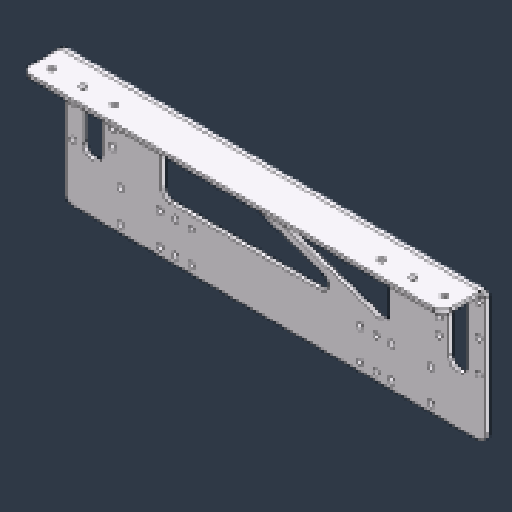
# Autodesk Inventor part: PLATE,MOUNT,DRIVE,ELEVATOR
Saved by Autodesk Inventor 2024.3 (Build 283343000, 343)
## iProperties
Category: _
Manager: _
Created: 2025-01-29
Part Number: PLATE,MOUNT,DRIVE,ELEVATOR
Checked By: 00
Engr Approved By: _
User Status: Work In Process
Material: Sheet Metal, Aluminum, 3003
Description: SHEET METAL (mm)
Document SubType Name: Sheet Metal
Mfg Approved By: John.Thibert
Designer: John.Thibert
Manufacturer: Standard
Standards Organization: Custom
Density: 2.73 g/cm^3
Sheet Metal Rule: Default
Appearance: Metal-AL-6061 (Flat)
Mass: 317.836 g
Surface Area: 810.801 cm^2
Volume: 116.424 cm^3
ILogicPurgeVersion: 2.2.20.20
OnSaveVersion: 3.4.3.0
OnSaveAssembly: COREAutomationManager
CN_MASS: 0.32
CL_runCount: 1
CN_SERVICEABLE: _
FIRST_DESCRIPTION: _
SECOND_DESCRIPTION: _
THIRD_DESCRIPTION: _
ModelCat: Uncategorized
MaterialName: Sheet Metal, Aluminum, 3003
Subject: _
Author: John.Thibert
Keywords: -
Revision Number: A
Autodesk Inventor part; units mm, degrees
ref_plane "YZ Plane" through (0, 0, 0) normal (1, 0, 0) x (0, 1, 0)
ref_plane "XZ Plane" through (0, 0, 0) normal (0, 1, 0) x (-1, 0, 0)
ref_plane "XY Plane" through (0, 0, 0) normal (0, 0, 1) x (1, 0, 0)
sketch "Sketch1" plane through (0, 0, 0) normal (0, 0, 1) x (1, 0, 0)
  line L0 (169.8625, -50.8) -> (-169.8625, -50.8)
  line L1 (-169.8625, -50.8) -> (-169.8625, 50.8)
  line L2 (-169.8625, 50.8) -> (169.8625, 50.8)
  line L3 (169.8625, 50.8) -> (169.8625, -50.8)
  line L4 (169.8625, -50.8) -> (-169.8625, 50.8) construction
  line L5 (-169.8625, -50.8) -> (169.8625, 50.8) construction
  point P0 (0, 0)
  dimension "d0" = 339.725
  dimension "d1" = 101.6
  measures "d0" distance of L1.end L2.end
  measures "d1" distance of L0.end L1.end
extrude "Plate1" add sketch "Sketch1" along normal mid plane 3.175
sketch "Sketch2" plane through (-169.8625, 55.5625, 6.35) normal (0, 1, 0) x (-1, 0, 0)
  line L0 (-339.725, 0) -> (0, 0)
  line L1 (0, 0) -> (0, 30.1625)
  line L2 (0, 30.1625) -> (-339.725, 30.1625)
  line L3 (-339.725, 30.1625) -> (-339.725, 0)
  constraints: 6 end point, 1 horizontal, 1 perpendicular, 1 vertical
edge flange "Flange1" height 38.1 angle 90 thickness 3.175 bend radius 4.7625 thickness toward (0, 1, 0) relief tear relief width 3.175 relief depth 1.5875 edges at (0, 50.8, 1.5875) wall of the first edge with corners at (169.8625, 55.5625, 6.35) (-169.8625, 55.5625, 6.35) (-169.8625, 55.5625, 36.5125) (169.8625, 55.5625, 36.5125)
bend "Bend1"
corner "Corner1"
sketch "Sketch3" plane through (0, 0, 1.5875) normal (0, 0, 1) x (1, 0, 0)
  line L0 (163.5252, -4.7625) -> (-163.5252, -4.7625) construction
  line L1 (-163.5252, -4.7625) -> (-163.5252, 46.0375) construction
  line L2 (-163.5252, 46.0375) -> (163.5252, 46.0375) construction
  line L3 (163.5252, 46.0375) -> (163.5252, -4.7625) construction
  line L4 (163.5252, -4.7625) -> (-163.5252, 46.0375) construction
  line L5 (-163.5252, -4.7625) -> (163.5252, 46.0375) construction
  line L6 (-237.8075, 0) -> (237.8075, 0) construction
  line L7 (0, 80.645) -> (0, -72.7075) construction
  line L8 (169.8625, 58.7375) -> (-169.8625, 58.7375) construction
  point P0 (0, 20.6375)
  point P1 (-163.5252, 20.6375)
  point P2 (163.5252, 20.6375)
  dimension "d13" = 327.0504
  dimension "d14" = 50.8
  dimension "d44" = 12.7
  constraints: 12 end point, 4 coincident, 4 midpoint, 2 parallel, 1 horizontal, 1 perpendicular, 1 point on line
  measures "d13" distance of L1.end L2.end
  measures "d14" distance of L0.end L1.end
  measures "d44" distance between parallel lines of L2 L8
hole "Hole1" at (-163.5252, 46.0375, 1.5875) at (163.5252, 46.0375, 1.5875) at (-163.5252, 20.6375, 1.5875) at (-163.5252, -4.7625, 1.5875) at (163.5252, 20.6375, 1.5875) at (163.5252, -4.7625, 1.5875) direction (0, 0, -1) diameter 5.1054 end through all clearance for "Flat Head Machine Screw (82)" size "#10" standard "Ansi Unified Screw Threads"
sketch "Sketch4" plane through (0, 0, 1.5875) normal (0, 0, 1) x (1, 0, 0)
  line L0 (95.25, -12.7) -> (-95.25, -12.7) construction
  line L1 (-95.25, -12.7) -> (-95.25, 50.8) construction
  line L2 (-95.25, 50.8) -> (95.25, 50.8) construction
  line L3 (95.25, 50.8) -> (95.25, -12.7) construction
  line L4 (95.25, -12.7) -> (-95.25, 50.8) construction
  line L5 (-95.25, -12.7) -> (95.25, 50.8) construction
  line L6 (-75.6848, 47.625) -> (92.075, 47.625)
  line L7 (92.075, 47.625) -> (92.075, -8.2949)
  line L8 (92.075, -8.2949) -> (-75.6848, 47.625)
  line L9 (-92.075, -9.525) -> (75.6848, -9.525)
  line L10 (75.6848, -9.525) -> (-92.075, 46.3949)
  line L11 (-92.075, 46.3949) -> (-92.075, -9.525)
  line L12 (-147.6375, -3.175) -> (-147.6375, 41.275) construction
  line L13 (-155.575, -3.175) -> (-155.575, 41.275)
  line L14 (-139.7, 41.275) -> (-139.7, -3.175)
  arc A0 (-155.575, -3.175) -> (-139.7, -3.175) centre (-147.6375, -3.175) ccw
  arc A1 (-139.7, 41.275) -> (-155.575, 41.275) centre (-147.6375, 41.275) ccw
  line L15 (0, 80.645) -> (0, -72.7075) construction
  line L16 (147.6375, -3.175) -> (147.6375, 41.275) construction
  line L17 (155.575, -3.175) -> (155.575, 41.275)
  line L18 (139.7, 41.275) -> (139.7, -3.175)
  arc A2 (139.7, -3.175) -> (155.575, -3.175) centre (147.6375, -3.175) ccw
  arc A3 (155.575, 41.275) -> (139.7, 41.275) centre (147.6375, 41.275) ccw
  line L19 (-147.6375, 19.05) -> (147.6375, 19.05) construction
  line L20 (-237.8075, 0) -> (237.8075, 0) construction
  line L21 (169.8625, 58.7375) -> (-169.8625, 58.7375) construction
  point P0 (0, 19.05)
  dimension "d22" = 63.5
  dimension "d23" = 190.5
  dimension "d24" = 3.175
  dimension "d25" = 3.175
  dimension "d29" = 7.9375
  dimension "d30" = 44.45
  dimension "d31" = 147.6375
  dimension "d45" = 39.6875
  constraints: 42 end point, 8 point on circle, 7 symmetric about line, 4 centre point, 4 midpoint, 4 tangent, 3 parallel, 3 perpendicular, 1 horizontal, 1 horizontal alignment, 1 vertical, 6 other
  measures "d22" distance of L0.end L1.end
  measures "d23" distance of L1.end L2.end
  measures "d24" distance between parallel lines of L0 L9
  measures "d25" distance between parallel lines of L2 L6
  measures "d29" radius of A1
  measures "d30" distance of L12.start L12.end
  measures "d31" distance between parallel lines of L12 L15
  measures "d45" distance between parallel lines of L19 L21
extrude "Cut1" cut sketch "Sketch4" against normal through all
sketch "Sketch6" plane through (0, 0, 1.5875) normal (0, 0, 1) x (1, 0, 0)
  line L0 (-93.6625, -19.05) -> (-93.6625, -44.45) construction
  line L1 (-169.8625, -50.8) -> (-169.8625, 50.8) construction
  point P0 (0, 0)
  dimension "d46" = 25.4
  dimension "d47" = 76.2
  dimension "d58" = 19.05
  constraints: 2 coincident, 2 end point, 1 vertical
  measures "d46" distance of L0.start L0.end
  measures "d47" distance between parallel lines of L1 L0
  measures "d58" vertical distance of point (-93.663, -19.05) point (0, 0)
hole "Hole2" at (-93.6625, -19.05, 1.5875) at (-93.6625, -44.45, 1.5875) direction (0, 0, -1) diameter 5.1054 end through all clearance for "Flat Head Machine Screw (82)" size "#10" standard "Ansi Unified Screw Threads"
pattern_linear "Rectangular Pattern1" count 2 spacing 31.75 along (-1, 0, 0) of "Hole2"
pattern_linear "Rectangular Pattern2" count 3 spacing 12.7 along (1, 0, 0) of "Hole2"
sketch "Sketch7" plane through (0, 0, 1.5875) normal (0, 0, 1) x (1, 0, 0)
  line L0 (-139.7, 41.275) -> (-139.7, -3.175) construction
  line L1 (-131.7625, 31.8516) -> (-131.7625, 6.4516) construction
  point P0 (0, 0)
  point P1 (-131.7625, 19.1516)
  dimension "d62" = 25.4
  dimension "d63" = 7.9375
  dimension "d64" = 19.1516
  constraints: 2 coincident, 2 end point, 1 midpoint, 1 vertical
  measures "d62" distance of L1.start L1.end
  measures "d63" distance between parallel lines of L0 L1
  measures "d64" vertical distance of point (0, 0) point (-131.763, 19.152)
hole "Hole3" at (-131.7625, 31.8516, 1.5875) at (-131.7625, 19.1516, 1.5875) at (-131.7625, 6.4516, 1.5875) direction (0, 0, -1) diameter 5.1054 end through all clearance for "Flat Head Machine Screw (82)" size "#10" standard "Ansi Unified Screw Threads"
sketch "Sketch8" plane through (-169.8625, 55.5625, 6.35) normal (0, -1, 0) x (1, 0, 0)
  line L0 (0, -4.7625) -> (339.725, -4.7625) construction
  line L1 (0, 30.1625) -> (0, 0) construction
  point P0 (169.8625, -6.35)
  point P1 (11.1125, 17.4625)
  dimension "d72" = 22.225
  dimension "d73" = 11.1125
  measures "d72" distance from line of point (11.113, 17.462) L0
  measures "d73" distance from line of point (11.113, 17.462) L1
mirror "Mirror1" about plane through (0, 0, 0) normal (1, 0, 0) of "Hole2", "Rectangular Pattern1", "Rectangular Pattern2", "Hole3"
hole "Hole4" at (-158.75, 55.5625, 23.8125) direction (0, 1, 0) diameter 5.1054 depth 3.175 tip angle 118 clearance for "Flat Head Machine Screw (82)" size "#10" standard "Ansi Unified Screw Threads"
pattern_linear "Rectangular Pattern3" count 3 spacing 25.4 along (1, 0, 0) of "Hole4"
mirror "Mirror2" about plane through (0, 0, 0) normal (1, 0, 0) of "Hole4", "Rectangular Pattern3"
fillet "Corner Round2" radius 6.35 10 edges at (169.8625, 57.15, 36.5125) (-169.8625, 57.15, 36.5125) (169.8625, -50.8, 0) (-169.8625, -50.8, 0) (-92.075, -9.525, 0) (75.6848, -9.525, 0) (-92.075, 46.3949, 0) (92.075, 47.625, 0) (-75.6848, 47.625, 0) (92.075, -8.2949, 0)
equation "\"d20\" = Thickness"
equation "\"d25\" = d24"
equation "\"d26\" = Thickness"
equation "\"d70\" = Thickness"
equation "\"d79\" = Thickness"
equation "\"d2\" = Thickness"
equation "\"d3\" = BendReliefWidth"
equation "\"d4\" = BendReliefDepth"
equation "\"d5\" = MinimumRemnant"
equation "\"d6\" = TransitionRadius"
equation "\"d9\" = BendRadius"
equation "\"d10\" = CornerReliefSize"
equation "\"d11\" = GapSize"
equation "\"d12\" = JacobiRadiusSize"
equation "\"BendRadius\" = 1.5 * Thickness"
equation "\"BendReliefWidth\" = Thickness"
equation "\"BendReliefDepth\" = 0.5 * Thickness"
equation "\"CornerReliefSize\" = 4 * Thickness"
equation "\"MinimumRemnant\" = 2 * Thickness"
equation "\"TransitionRadius\" = BendRadius"
equation "\"JacobiRadiusSize\" = BendRadius"
equation "\"GapSize\" = Thickness"
equation "\"Thickness\" = 3.175"
body "Solid1"
